Autodesk Fusion 360 part; units mm, degrees
(part 2 of 3)
  line L471 (-71.7601, 16.325) -> (-71.7601, 17.325)
  line L472 (-74.2601, 12.625) -> (-74.2601, 11.625)
  line L473 (-71.1601, 14.475) -> (-70.1601, 13.225) construction
  line L474 (-74.2601, 12.625) -> (-74.2601, 11.625)
  line L475 (-74.8601, 14.475) -> (-75.8601, 13.225) construction
  line L476 (-74.2601, 12.625) -> (-74.2601, 11.625)
  line L477 (-74.2601, 17.325) -> (-73.0101, 16.325) construction
  line L478 (-71.7601, 11.625) -> (-71.7601, 12.625)
  line L479 (-70.1601, 15.725) -> (-71.1601, 15.725)
  line L480 (-74.2601, 11.625) -> (-73.0101, 12.625) construction
  line L481 (-71.7601, 11.625) -> (-71.7601, 12.625)
  line L482 (-75.8601, 15.725) -> (-74.8601, 15.725)
  line L483 (-74.2601, 12.625) -> (-74.2601, 11.625)
  line L484 (-74.8601, 14.475) -> (-75.8601, 13.225) construction
  line L485 (-71.1601, 13.225) -> (-70.1601, 13.225)
  line L486 (-75.8601, 15.725) -> (-74.8601, 15.725)
  line L487 (-74.2601, 12.625) -> (-74.2601, 11.625)
  line L488 (-74.2601, 12.625) -> (-74.2601, 11.625)
  line L489 (-74.2601, 12.625) -> (-74.2601, 11.625)
  line L490 (-74.2601, 17.325) -> (-73.0101, 16.325) construction
  line L491 (-70.1601, 15.725) -> (-71.1601, 15.725)
  line L492 (-75.8601, 15.725) -> (-74.8601, 15.725)
  line L493 (-74.8601, 13.225) -> (-75.8601, 13.225)
  line L494 (-74.8601, 13.225) -> (-75.8601, 13.225)
  line L495 (-75.8601, 15.725) -> (-74.8601, 15.725)
  line L496 (-71.1601, 13.225) -> (-70.1601, 13.225)
  line L497 (-74.8601, 14.475) -> (-75.8601, 13.225) construction
  line L498 (-71.7601, 16.325) -> (-71.7601, 17.325)
  line L499 (-71.1601, 14.475) -> (-70.1601, 13.225) construction
  line L500 (-70.1601, 15.725) -> (-71.1601, 15.725)
  line L501 (-71.1601, 13.225) -> (-70.1601, 13.225)
  line L502 (-74.2601, 17.325) -> (-73.0101, 16.325) construction
  line L503 (-71.1601, 14.475) -> (-70.1601, 13.225) construction
  line L504 (-71.1601, 14.475) -> (-70.1601, 13.225) construction
  line L505 (-74.2601, 17.325) -> (-73.0101, 16.325) construction
  line L506 (-74.2601, 11.625) -> (-73.0101, 12.625) construction
  line L507 (-74.2601, 17.325) -> (-74.2601, 16.325)
  line L508 (-74.8601, 13.225) -> (-75.8601, 13.225)
  line L509 (-70.1601, 15.725) -> (-71.1601, 15.725)
  line L510 (-74.8601, 14.475) -> (-75.8601, 13.225) construction
  line L511 (-71.7601, 11.625) -> (-71.7601, 12.625)
  line L512 (-71.7601, 16.325) -> (-71.7601, 17.325)
  line L513 (-71.7601, 16.325) -> (-71.7601, 17.325)
  line L514 (-71.7601, 11.625) -> (-71.7601, 12.625)
  line L515 (-70.1601, 15.725) -> (-71.1601, 15.725)
  line L516 (-74.2601, 12.625) -> (-74.2601, 11.625)
  line L517 (-74.8601, 13.225) -> (-75.8601, 13.225)
  line L518 (-74.2601, 17.325) -> (-74.2601, 16.325)
  line L519 (-71.7601, 11.625) -> (-71.7601, 12.625)
  line L520 (-74.2601, 17.325) -> (-74.2601, 16.325)
  line L521 (-70.1601, 15.725) -> (-71.1601, 15.725)
  line L522 (-71.1601, 13.225) -> (-70.1601, 13.225)
  line L523 (-71.1601, 13.225) -> (-70.1601, 13.225)
  line L524 (-74.2601, 11.625) -> (-73.0101, 12.625) construction
  line L525 (-70.1601, 15.725) -> (-71.1601, 15.725)
  line L526 (-74.2601, 17.325) -> (-74.2601, 16.325)
  line L527 (-71.7601, 11.625) -> (-71.7601, 12.625)
  line L528 (-71.1601, 13.225) -> (-70.1601, 13.225)
  line L529 (-71.1601, 13.225) -> (-70.1601, 13.225)
  line L530 (-70.1601, 15.725) -> (-71.1601, 14.475) construction
  line L531 (-75.8601, 15.725) -> (-74.8601, 15.725)
  line L532 (-74.2601, 12.625) -> (-74.2601, 11.625)
  line L533 (-74.8601, 13.225) -> (-75.8601, 13.225)
  line L534 (-70.1601, 15.725) -> (-71.1601, 14.475) construction
  line L535 (-75.8601, 15.725) -> (-74.8601, 15.725)
  line L536 (-70.1601, 13.225) -> (-70.1601, 15.725)
  line L537 (-74.8601, 16.325) -> (-74.8601, 12.625)
  line L538 (-70.1601, 13.225) -> (-70.1601, 15.725)
  line L539 (-74.8601, 14.475) -> (-75.8601, 13.225) construction
  line L540 (-74.8601, 14.475) -> (-75.8601, 13.225) construction
  line L541 (-74.2601, 12.625) -> (-74.2601, 11.625)
  line L542 (-75.8601, 15.725) -> (-74.8601, 15.725)
  line L543 (-74.2601, 17.325) -> (-74.2601, 16.325)
  line L544 (-74.2601, 12.625) -> (-74.2601, 11.625)
  line L545 (-74.2601, 12.625) -> (-74.2601, 11.625)
  line L546 (-74.2601, 17.325) -> (-74.2601, 16.325)
  line L547 (-70.1601, 13.225) -> (-70.1601, 15.725)
  line L548 (-75.8601, 15.725) -> (-74.8601, 15.725)
  line L549 (-74.8601, 16.325) -> (-74.8601, 12.625)
  line L550 (-74.2601, 17.325) -> (-73.0101, 16.325) construction
  line L551 (-74.8601, 14.475) -> (-75.8601, 13.225) construction
  line L552 (-74.2601, 17.325) -> (-74.2601, 16.325)
  line L553 (-74.2601, 11.625) -> (-73.0101, 12.625) construction
  line L554 (-70.1601, 15.725) -> (-71.1601, 14.475) construction
  line L555 (-71.1601, 12.625) -> (-71.1601, 16.325)
  line L556 (-74.8601, 13.225) -> (-75.8601, 13.225)
  line L557 (-71.1601, 12.625) -> (-71.1601, 16.325)
  line L558 (-74.2601, 12.625) -> (-74.2601, 11.625)
  line L559 (-70.1601, 13.225) -> (-70.1601, 15.725)
  line L560 (-74.8601, 13.225) -> (-75.8601, 13.225)
  line L561 (-71.1601, 12.625) -> (-71.1601, 16.325)
  line L562 (-70.1601, 15.725) -> (-71.1601, 14.475) construction
  line L563 (-74.8601, 14.475) -> (-75.8601, 13.225) construction
  line L564 (-74.2601, 12.625) -> (-74.2601, 11.625)
  line L565 (-74.2601, 11.625) -> (-73.0101, 12.625) construction
  line L566 (-74.2601, 17.325) -> (-74.2601, 16.325)
  line L567 (-74.2601, 11.625) -> (-73.0101, 12.625) construction
  line L568 (-70.1601, 13.225) -> (-70.1601, 15.725)
  line L569 (-70.1601, 13.225) -> (-70.1601, 15.725)
  line L570 (-74.2601, 17.325) -> (-73.0101, 16.325) construction
  line L571 (-74.8601, 13.225) -> (-75.8601, 13.225)
  line L572 (3.5, 7.3942) -> (-58, 7.3942)
  line L573 (-58, 7.3942) -> (-58, 35.3942)
  line L574 (-58, 35.3942) -> (3.5, 35.3942)
  line L575 (3.5, 35.3942) -> (3.5, 7.3942)
  point P0 (-73.0101, 27.475)
  point P1 (-73.0351, 14.5)
  point P2 (-73.0101, 27.475)
  point P3 (-73.0101, 27.475)
  point P4 (-73.0101, 27.475)
  point P5 (-73.0101, 27.475)
  point P6 (-73.0101, 27.475)
  point P7 (-73.0101, 27.475)
  point P8 (-73.0101, 27.475)
  point P9 (-73.0101, 14.475)
  point P10 (-73.0101, 14.475)
  point P11 (-73.0101, 14.475)
  point P12 (-73.0101, 14.475)
  point P13 (-73.0101, 14.475)
  point P14 (-73.0101, 14.475)
  point P15 (-73.0101, 14.475)
  point P16 (-73.0101, 14.475)
  dimension "d66" = -3
  dimension "d68" = 5
  dimension "d69" = 5
  dimension "d70" = 5
  dimension "d71" = 5
  dimension "d72" = 2
  dimension "d74" = 2
  dimension "d75" = 2
  dimension "d76" = 2
  dimension "d77" = 2
  dimension "d88" = 0.3
  dimension "d122" = 3.7
  dimension "d123" = 3.7
  dimension "d134" = 3.7
  dimension "d135" = 3.7
  dimension "d136" = 3.7
  dimension "d137" = 3.7
  dimension "d138" = 3.7
  dimension "d139" = 3.7
  dimension "d140" = 3.7
  dimension "d141" = 3.7
  dimension "d142" = 3.7
  dimension "d143" = 3.7
  dimension "d144" = 3.7
  dimension "d145" = 3.7
  dimension "d146" = 3.7
  dimension "d147" = 3.7
  dimension "d148" = 3.7
  dimension "d149" = 3.7
  dimension "d150" = 3.7
  dimension "d151" = 3.7
  dimension "d152" = 3.7
  dimension "d153" = 3.7
  dimension "d154" = 3.7
  dimension "d155" = 3.7
  dimension "d156" = 3.7
  dimension "d157" = 3.7
  dimension "d158" = 3.7
  dimension "d159" = 3.7
  dimension "d160" = 3.7
  dimension "d161" = 3.7
  dimension "d162" = 3.7
  dimension "d163" = 3.7
  constraint tangent L18 A12
  constraint tangent L17 A12
  constraint tangent L17 A13
  constraint tangent L16 A13
  constraint tangent L19 A14
  constraint tangent L16 A14
  constraint tangent L18 A15
  constraint tangent L19 A15
  constraint tangent L27 A20
  constraint tangent L26 A20
  constraint tangent L25 A21
  constraint tangent L26 A21
  constraint tangent L24 A22
  constraint tangent L25 A22
  constraint tangent L24 A23
  constraint tangent L27 A23
  constraint horizontal L33
  constraint vertical L34
  constraint horizontal L35
  constraint vertical L36
  constraint coincident L31.end L34.end
  constraint coincident L5.end L6.start
  constraint horizontal L37
  constraint vertical L38
  constraint horizontal L39
  constraint vertical L40
  constraint coincident L4.start L7.end
  constraint coincident L31.start L35.end
  constraint coincident L42 L55.start
  constraint coincident L5 L40.start
  constraint coincident L7 L55.end
  constraint perpendicular L50 L56
  constraint coincident L50 L56.end
  constraint coincident L49 L57.end
  constraint perpendicular L49 L57
  constraint horizontal L58
  constraint perpendicular L58 L59
  constraint parallel L58 L60
  constraint parallel L59 L61
  constraint coincident L62 P8
  constraint coincident L63 P8
  constraint horizontal L64
  constraint perpendicular L64 L68
  constraint parallel L65 L68
  constraint midpoint L60 L66.end
  constraint coincident L60 L68.end
  constraint coincident L60 L65.start
  constraint horizontal L73
  constraint midpoint L59 L70.end
  constraint coincident L59 L72.start
  constraint coincident L59 L73.end
  constraint horizontal L76
  constraint midpoint L61 L75.end
  constraint coincident L61 L76.end
  constraint coincident L61 L77.start
  constraint horizontal L79
  constraint perpendicular L79 L82
  constraint parallel L80 L82
  constraint midpoint L58 L81.end
  constraint coincident L58 L82.end
  constraint coincident L58 L80.start
  constraint horizontal L85
  constraint perpendicular L85 L86
  constraint parallel L84 L86
  constraint horizontal L89
  constraint horizontal L117
  constraint perpendicular L113 L117
  constraint parallel L91 L117
  constraint parallel L110 L113
  constraint coincident P8 L116
  constraint coincident P8 L90
  constraint horizontal L118
  constraint perpendicular L100 L118
  constraint parallel L99 L100
  constraint midpoint L66.end L91
  constraint coincident L68.end L91
  constraint coincident L65.start L91
  constraint horizontal L106
  constraint midpoint L70.end L113
  constraint coincident L72.start L113
  constraint coincident L73.end L113
  constraint horizontal L104
  constraint midpoint L75.end L110
  constraint coincident L76.end L110
  constraint coincident L77.start L110
  constraint horizontal L115
  constraint perpendicular L105 L115
  constraint parallel L105 L111
  constraint midpoint L81.end L117
  constraint coincident L82.end L117
  constraint coincident L80.start L117
  constraint horizontal L119
  constraint perpendicular L114 L119
  constraint parallel L96 L114
  constraint horizontal L102
  constraint midpoint L41 L122.start
  constraint midpoint L43 L122.end
  constraint midpoint L42 L123.start
  constraint midpoint L44 L123.end
  constraint horizontal L158
  constraint perpendicular L151 L158
  constraint parallel L138 L158
  constraint parallel L129 L151
  constraint coincident P8 L164
  constraint coincident P8 L163
  constraint horizontal L140
  constraint perpendicular L140 L149
  constraint parallel L142 L149
  constraint midpoint L66.end L138
  constraint coincident L68.end L138
  constraint coincident L65.start L138
  constraint horizontal L125
  constraint midpoint L70.end L151
  constraint coincident L72.start L151
  constraint coincident L73.end L151
  constraint horizontal L128
  constraint midpoint L75.end L129
  constraint coincident L76.end L129
  constraint coincident L77.start L129
  constraint horizontal L143
  constraint perpendicular L143 L178
  constraint parallel L141 L178
  constraint midpoint L81.end L158
  constraint coincident L82.end L158
  constraint coincident L80.start L158
  constraint horizontal L137
  constraint perpendicular L137 L169
  constraint parallel L169 L186
  constraint horizontal L182
  constraint horizontal L165
  constraint perpendicular L127 L165
  constraint parallel L159 L165
  constraint parallel L127 L174
  constraint coincident P8 L162
  constraint coincident P8 L161
  constraint horizontal L133
  constraint perpendicular L133 L155
  constraint parallel L155 L181
  constraint midpoint L66.end L159
  constraint coincident L68.end L159
  constraint coincident L65.start L159
  constraint horizontal L176
  constraint midpoint L70.end L127
  constraint coincident L72.start L127
  constraint coincident L73.end L127
  constraint horizontal L152
  constraint midpoint L75.end L174
  constraint coincident L76.end L174
  constraint coincident L77.start L174
  constraint horizontal L134
  constraint perpendicular L134 L180
  constraint parallel L157 L180
  constraint midpoint L81.end L165
  constraint coincident L82.end L165
  constraint coincident L80.start L165
  constraint horizontal L136
  constraint perpendicular L124 L136
  constraint parallel L124 L148
  constraint horizontal L175
  constraint horizontal L219
  constraint perpendicular L197 L219
  constraint parallel L219 L226
  constraint parallel L197 L198
  constraint coincident P8 L212
  constraint coincident P8 L215
  constraint horizontal L191
  constraint perpendicular L191 L283
  constraint parallel L252 L283
  constraint midpoint L66.end L226
  constraint coincident L68.end L226
  constraint coincident L65.start L226
  constraint horizontal L262
  constraint midpoint L70.end L197
  constraint coincident L72.start L197
  constraint coincident L73.end L197
  constraint horizontal L246
  constraint midpoint L75.end L198
  constraint coincident L76.end L198
  constraint coincident L77.start L198
  constraint horizontal L216
  constraint perpendicular L216 L248
  constraint parallel L238 L248
  constraint midpoint L81.end L219
  constraint coincident L82.end L219
  constraint coincident L80.start L219
  constraint horizontal L221
  constraint perpendicular L221 L258
  constraint parallel L251 L258
  constraint horizontal L291
  constraint horizontal L218
  constraint perpendicular L218 L228
  constraint parallel L218 L220
  constraint parallel L196 L228
  constraint coincident P8 L217
  constraint coincident P8 L213
  constraint horizontal L225
  constraint perpendicular L225 L242
  constraint parallel L242 L300
  constraint midpoint L66.end L220
  constraint coincident L68.end L220
  constraint coincident L65.start L220
  constraint horizontal L247
  constraint midpoint L70.end L228
  constraint coincident L72.start L228
  constraint coincident L73.end L228
  constraint horizontal L268
  constraint midpoint L75.end L196
  constraint coincident L76.end L196
  constraint coincident L77.start L196
  constraint horizontal L188
  constraint perpendicular L188 L233
  constraint parallel L233 L264
  constraint midpoint L81.end L218
  constraint coincident L82.end L218
  constraint coincident L80.start L218
  constraint horizontal L224
  constraint perpendicular L224 L260
  constraint parallel L260 L314
  constraint horizontal L234
  constraint horizontal L194
  constraint perpendicular L194 L239
  constraint parallel L194 L206
  constraint parallel L239 L261
  constraint coincident P8 L203
  constraint coincident P8 L202
  constraint horizontal L214
  constraint perpendicular L214 L292
  constraint parallel L292 L299
  constraint midpoint L66.end L206
  constraint coincident L68.end L206
  constraint coincident L65.start L206
  constraint horizontal L280
  constraint midpoint L70.end L239
  constraint coincident L72.start L239
  constraint coincident L73.end L239
  constraint horizontal L296
  constraint midpoint L75.end L261
  constraint coincident L76.end L261
  constraint coincident L77.start L261
  constraint horizontal L192
  constraint perpendicular L192 L272
  constraint parallel L272 L276
  constraint midpoint L81.end L194
  constraint coincident L82.end L194
  constraint coincident L80.start L194
  constraint horizontal L193
  constraint perpendicular L193 L290
  constraint parallel L278 L290
  constraint horizontal L282
  constraint horizontal L195
  constraint perpendicular L195 L229
  constraint parallel L195 L210
  constraint parallel L229 L243
  constraint coincident P8 L204
  constraint coincident P8 L201
  constraint horizontal L207
  constraint perpendicular L207 L293
  constraint parallel L293 L312
  constraint midpoint L66.end L210
  constraint coincident L68.end L210
  constraint coincident L65.start L210
  constraint horizontal L240
  constraint midpoint L70.end L229
  constraint coincident L72.start L229
  constraint coincident L73.end L229
  constraint horizontal L286
  constraint midpoint L75.end L243
  constraint coincident L76.end L243
  constraint coincident L77.start L243
  constraint horizontal L200
  constraint perpendicular L200 L304
  constraint parallel L294 L304
  constraint midpoint L81.end L195
  constraint coincident L82.end L195
  constraint coincident L80.start L195
  constraint horizontal L205
  constraint perpendicular L205 L288
  constraint parallel L285 L288
  constraint horizontal L311
  constraint horizontal L348
  constraint perpendicular L348 L357
  constraint parallel L317 L348
  constraint parallel L357 L369
  constraint coincident P16 L340
  constraint coincident P16 L327
  constraint horizontal L423
  constraint perpendicular L423 L514
  constraint parallel L488 L514
  constraint midpoint L319.end L317
  constraint coincident L431.end L317
  constraint coincident L440.start L317
  constraint horizontal L548
  constraint midpoint L351.end L357
  constraint coincident L493.start L357
  constraint coincident L482.end L357
  constraint horizontal L515
  constraint midpoint L361.end L369
  constraint coincident L433.end L369
  constraint coincident L435.start L369
  constraint horizontal L346
  constraint perpendicular L346 L546
  constraint parallel L463 L546
  constraint midpoint L326.end L348
  constraint coincident L507.end L348
  constraint coincident L429.start L348
  constraint horizontal L337
  constraint perpendicular L337 L481
  constraint parallel L481 L564
  constraint horizontal L525
  constraint horizontal L424
  constraint perpendicular L385 L424
  constraint parallel L338 L424
  constraint parallel L350 L385
  constraint coincident P16 L341
  constraint coincident P16 L342
  constraint horizontal L344
  constraint perpendicular L344 L519
  constraint parallel L519 L544
  constraint midpoint L319.end L338
  constraint coincident L431.end L338
  constraint coincident L440.start L338
  constraint horizontal L542
  constraint midpoint L351.end L385
  constraint coincident L493.start L385
  constraint coincident L482.end L385
  constraint horizontal L443
  constraint midpoint L361.end L350
  constraint coincident L433.end L350
  constraint coincident L435.start L350
  constraint horizontal L425
  constraint perpendicular L425 L566
  constraint parallel L512 L566
  constraint midpoint L326.end L424
  constraint coincident L507.end L424
  constraint coincident L429.start L424
  constraint horizontal L426
  constraint perpendicular L426 L527
  constraint parallel L527 L532
  constraint horizontal L509
  constraint horizontal L427
  constraint perpendicular L353 L427
  constraint parallel L325 L427
  constraint parallel L353 L368
  constraint coincident P16 L334
  constraint coincident P16 L339
  constraint horizontal L345
  constraint perpendicular L345 L444
  constraint parallel L444 L545
  constraint midpoint L319.end L325
  constraint coincident L431.end L325
  constraint coincident L440.start L325
  constraint horizontal L531
  constraint midpoint L351.end L353
  constraint coincident L493.start L353
  constraint coincident L482.end L353
  constraint horizontal L500
  constraint midpoint L361.end L368
  constraint coincident L433.end L368
  constraint coincident L435.start L368
  constraint horizontal L320
  constraint perpendicular L320 L543
  constraint parallel L498 L543
  constraint midpoint L326.end L427
  constraint coincident L507.end L427
  constraint coincident L429.start L427
  constraint horizontal L343
  constraint perpendicular L343 L478
  constraint parallel L478 L558
  constraint horizontal L479
  constraint horizontal L347
  constraint perpendicular L347 L366
  constraint parallel L329 L347
  constraint parallel L360 L366
  constraint coincident P16 L322
  constraint coincident P16 L321
  constraint horizontal L333
  constraint perpendicular L333 L511
  constraint parallel L483 L511
  constraint midpoint L319.end L329
  constraint coincident L431.end L329
  constraint coincident L440.start L329
  constraint horizontal L535
  constraint midpoint L351.end L366
  constraint coincident L493.start L366
  constraint coincident L482.end L366
  constraint horizontal L521
  constraint midpoint L361.end L360
  constraint coincident L433.end L360
  constraint coincident L435.start L360
  constraint horizontal L328
  constraint perpendicular L328 L552
  constraint parallel L513 L552
  constraint midpoint L326.end L347
  constraint coincident L507.end L347
  constraint coincident L429.start L347
  constraint horizontal L316
  constraint perpendicular L316 L436
  constraint parallel L436 L541
  constraint horizontal L491
  constraint horizontal L409
  constraint perpendicular L409 L549
  constraint parallel L402 L409
  constraint parallel L549 L555
  constraint coincident P16 L406
  constraint coincident P16 L394
  constraint horizontal L412
  constraint perpendicular L412 L459
  constraint parallel L459 L474
  constraint midpoint L319.end L402
  constraint coincident L431.end L402
  constraint coincident L440.start L402
  constraint horizontal L482
  constraint midpoint L351.end L549
  constraint coincident L493.start L549
  constraint coincident L482.end L549
  constraint horizontal L434
  constraint midpoint L361.end L555
  constraint coincident L433.end L555
  constraint coincident L435.start L555
  constraint horizontal L405
  constraint perpendicular L405 L526
  constraint parallel L462 L526
  constraint midpoint L326.end L409
  constraint coincident L507.end L409
  constraint coincident L429.start L409
  constraint horizontal L330
  constraint perpendicular L330 L449
  constraint parallel L449 L476
  constraint horizontal L453
  constraint horizontal L392
  constraint perpendicular L359 L392
  constraint parallel L392 L395
  constraint parallel L352 L359
  constraint coincident P16 L413
  constraint coincident P16 L404
  constraint horizontal L318
  constraint perpendicular L318 L458
  constraint parallel L458 L489
  constraint midpoint L319.end L395
  constraint coincident L431.end L395
  constraint coincident L440.start L395
  constraint horizontal L492
  constraint midpoint L351.end L359
  constraint coincident L493.start L359
  constraint coincident L482.end L359
  constraint horizontal L438
  constraint midpoint L361.end L352
  constraint coincident L433.end L352
  constraint coincident L435.start L352
  constraint horizontal L408
  constraint perpendicular L408 L507
  constraint parallel L471 L507
  constraint midpoint L326.end L392
  constraint coincident L507.end L392
  constraint coincident L429.start L392
  constraint horizontal L421
  constraint perpendicular L421 L441
  constraint parallel L441 L516
  constraint horizontal L433
  constraint horizontal L397
  constraint perpendicular L386 L397
  constraint parallel L397 L416
  constraint parallel L386 L557
  constraint coincident P16 L414
  constraint coincident P16 L389
  constraint horizontal L401
  constraint perpendicular L401 L437
  constraint parallel L437 L472
  constraint midpoint L319.end L416
  constraint coincident L431.end L416
  constraint coincident L440.start L416
  constraint horizontal L495
  constraint midpoint L351.end L386
  constraint coincident L493.start L386
  constraint coincident L482.end L386
  constraint horizontal L461
  constraint midpoint L361.end L557
  constraint coincident L433.end L557
  constraint coincident L435.start L557
  constraint horizontal L399
  constraint perpendicular L399 L518
  constraint parallel L430 L518
  constraint midpoint L326.end L397
  constraint coincident L507.end L397
  constraint coincident L429.start L397
  constraint horizontal L422
  constraint perpendicular L422 L457
  constraint parallel L457 L487
  constraint horizontal L448
  constraint horizontal L420
  constraint perpendicular L420 L537
  constraint parallel L400 L420
  constraint parallel L537 L561
  constraint coincident P16 L390
  constraint coincident P16 L410
  constraint horizontal L403
  constraint perpendicular L403 L467
  constraint parallel L440 L467
  constraint midpoint L319.end L400
  constraint coincident L431.end L400
  constraint coincident L440.start L400
  constraint horizontal L486
  constraint midpoint L351.end L537
  constraint coincident L493.start L537
  constraint coincident L482.end L537
  constraint horizontal L460
  constraint midpoint L361.end L561
  constraint coincident L433.end L561
  constraint coincident L435.start L561
  constraint horizontal L418
  constraint perpendicular L418 L520
  constraint parallel L429 L520
  constraint midpoint L326.end L420
  constraint coincident L507.end L420
  constraint coincident L429.start L420
  constraint horizontal L393
  constraint perpendicular L393 L431
  constraint parallel L431 L466
  constraint horizontal L470
  measures "d68" radius of A12
  measures "d69" radius of A13
  measures "d70" radius of A14
  measures "d71" radius of A15
  measures "d74" radius of A20
  measures "d75" radius of A21
  measures "d76" radius of A22
  measures "d77" radius of A23
  measures "d122" distance of L59.end L60.end
  measures "d123" distance of L58.end L59.end
  measures "d134" distance of L60.end L59.end
  measures "d135" distance of L58.end L59.end
  measures "d136" distance of L60.end L59.end
  measures "d137" distance of L58.end L59.end
  measures "d138" distance of L60.end L59.end
  measures "d139" distance of L58.end L59.end
  measures "d140" distance of L60.end L59.end
  measures "d141" distance of L58.end L59.end
  measures "d142" distance of L60.end L59.end
  measures "d143" distance of L58.end L59.end
  measures "d144" distance of L60.end L59.end
  measures "d145" distance of L59.end L58.end
  measures "d146" distance of L59.end L60.end
  measures "d147" distance of L59.end L58.end
  measures "d148" distance of L317.end L317.start
  measures "d149" distance of L321.start L317.start
  measures "d150" distance of L317.end L317.start
  measures "d151" distance of L321.start L317.start
  measures "d152" distance of L317.end L317.start
  measures "d153" distance of L317.start L321.start
  measures "d154" distance of L317.start L317.end
  measures "d155" distance of L317.start L321.start
  measures "d156" distance of L317.start L317.end
  measures "d157" distance of L317.start L321.start
  measures "d158" distance of L317.end L317.start
  measures "d159" distance of L321.start L317.start
  measures "d160" distance of L317.end L317.start
  measures "d161" distance of L317.start L321.start
  measures "d162" distance of L317.start L317.end
  measures "d163" distance of L317.start L321.start
extrude "Extrude10" cut sketch "Sketch4" against normal blind 0.5 contours A8 L12 A9 L13 A10 L14 A11 L15 | L16 L17 L18 L19 A12 A13 A14 A15 | L24 L25 L26 L27 A20 A21 A22 A23 bodies 2
extrude "Extrude11" add sketch "Sketch4" against normal blind 0.5 separate body contours A0 L0 A1 L1 A2 L2 A3 L3 | A8 L12 A9 L13 A10 L14 A11 L15 | L16 L17 L18 L19 A12 A13 A14 A15 makes body 3 at (-1.3333, 56.6667, 20) makes body 4 at (30.3333, -9.8109, 20)
extrude "Extrude12" add sketch "Sketch1" along normal blind 14 from surface at 2 separate body contours L0 L1 L2 L3 A0 A1 A2 A3 L59 L63 L68 L72 makes body 5
extrude "Extrude13" add sketch "Sketch4" against normal blind 2 from surface at -0.5 separate body contours L24 L25 L26 L27 A20 A21 A22 A23 makes body 6
extrude "Extrude14" add sketch "Sketch4" against normal blind 2 from surface at -4 separate body contours L4 L5 L7 L28 L29 L30 L38 L39 L40 L49 L50 L52 L53 L54 L56 L57 | L4 L5 L7 L28 L29 L30 L31 L35 L37 L38 L39 L40 | L45 L46 L47 L48 | L58 L59 L60 L61 L91 L110 L113 L117 L127 L129 L138 L151 L158 L159 L165 L174 L194 L195 L196 L197 L198 L206 L210 L218 L219 L220 L226 L228 L229 L239 L243 L261 | L58 L79 L80 L82 L105 L111 L115 L117 L134 L141 L143 L157 L158 L165 L178 L180 L188 L192 L194 L195 L200 L216 L218 L219 L233 L238 L248 L264 L272 L276 L294 L304 | L61 L74 L76 L77 L87 L88 L89 L92 L97 L102 L104 L107 L109 L110 L128 L129 L131 L150 L152 L170 L172 L173 L174 L175 L177 L182 L184 L187 L196 L198 L227 L230 L232 L234 L237 L241 L243 L246 L250 L254 L256 L261 L266 L268 L282 L286 L289 L291 L296 L297 L298 L301 L303 L306 L307 L311 | L59 L69 L72 L73 L103 L106 L108 L113 L125 L127 L130 L132 L151 L160 L167 L176 L197 L228 L229 L236 L239 L240 L247 L253 L255 L262 L270 L271 L279 L280 L284 L295 | L60 L64 L65 L68 L84 L85 L86 L91 L96 L99 L100 L114 L118 L119 L124 L133 L136 L137 L138 L140 L142 L148 L149 L155 L159 L169 L181 L186 L191 L193 L205 L206 L207 L210 L214 L220 L221 L224 L225 L226 L242 L251 L252 L258 L260 L278 L283 L285 L288 L290 L292 L293 L299 L300 L312 L314 makes body 7
extrude "Extrude15" add sketch "Sketch4" against normal blind 2 from surface at -4 separate body contours L5 L6 L7 L28 L29 L31 L32 L33 L34 L35 L36 L37 | L5 L6 L7 L28 L29 L32 L33 L34 L36 L49 L50 L51 L56 L57 | L41 L42 L43 L44 | L316 L317 L318 L325 L329 L330 L333 L337 L338 L343 L344 L345 L393 L395 L400 L401 L402 L403 L412 L416 L421 L422 L423 L426 L431 L436 L437 L440 L441 L444 L449 L457 L458 L459 L466 L467 L472 L474 L476 L478 L481 L483 L487 L488 L489 L511 L514 L516 L519 L527 L532 L541 L544 L545 L558 L564 | L317 L325 L329 L338 L347 L348 L350 L352 L353 L357 L359 L360 L366 L368 L369 L385 L386 L392 L395 L397 L400 L402 L409 L416 L420 L424 L427 L537 L549 L555 L557 L561 | L353 L355 L357 L358 L359 L364 L366 L367 L371 L375 L378 L383 L385 L386 L482 L486 L492 L493 L494 L495 L508 L517 L531 L533 L535 L537 L542 L548 L549 L556 L560 L571 | L349 L350 L352 L356 L360 L362 L365 L368 L369 L377 L379 L380 L384 L388 L391 L433 L434 L435 L438 L439 L443 L445 L446 L447 L448 L450 L451 L452 L453 L454 L460 L461 L470 L479 L485 L491 L496 L500 L501 L509 L515 L521 L522 L523 L525 L528 L529 L536 L538 L547 L555 L557 L559 L561 L568 L569 | L320 L328 L346 L347 L348 L392 L397 L399 L405 L408 L409 L418 L420 L424 L425 L427 L429 L430 L462 L463 L471 L498 L507 L512 L513 L518 L520 L526 L543 L546 L552 L566 makes body 8
extrude "Extrude16" add sketch "Sketch4" against normal blind 5 from surface at 1 contours L41 L42 L43 L44 | L316 L317 L318 L325 L329 L330 L333 L337 L338 L343 L344 L345 L393 L395 L400 L401 L402 L403 L412 L416 L421 L422 L423 L426 L431 L436 L437 L440 L441 L444 L449 L457 L458 L459 L466 L467 L472 L474 L476 L478 L481 L483 L487 L488 L489 L511 L514 L516 L519 L527 L532 L541 L544 L545 L558 L564 | L317 L325 L329 L338 L347 L348 L350 L352 L353 L357 L359 L360 L366 L368 L369 L385 L386 L392 L395 L397 L400 L402 L409 L416 L420 L424 L427 L537 L549 L555 L557 L561 | L353 L355 L357 L358 L359 L364 L366 L367 L371 L375 L378 L383 L385 L386 L482 L486 L492 L493 L494 L495 L508 L517 L531 L533 L535 L537 L542 L548 L549 L556 L560 L571 | L349 L350 L352 L356 L360 L362 L365 L368 L369 L377 L379 L380 L384 L388 L391 L433 L434 L435 L438 L439 L443 L445 L446 L447 L448 L450 L451 L452 L453 L454 L460 L461 L470 L479 L485 L491 L496 L500 L501 L509 L515 L521 L522 L523 L525 L528 L529 L536 L538 L547 L555 L557 L559 L561 L568 L569 | L320 L328 L346 L347 L348 L392 L397 L399 L405 L408 L409 L418 L420 L424 L425 L427 L429 L430 L462 L463 L471 L498 L507 L512 L513 L518 L520 L526 L543 L546 L552 L566 bodies 8
extrude "Extrude17" add sketch "Sketch4" against normal blind 5 from surface at 1 contours L45 L46 L47 L48 | L58 L59 L60 L61 L91 L110 L113 L117 L127 L129 L138 L151 L158 L159 L165 L174 L194 L195 L196 L197 L198 L206 L210 L218 L219 L220 L226 L228 L229 L239 L243 L261 | L58 L79 L80 L82 L105 L111 L115 L117 L134 L141 L143 L157 L158 L165 L178 L180 L188 L192 L194 L195 L200 L216 L218 L219 L233 L238 L248 L264 L272 L276 L294 L304 | L61 L74 L76 L77 L87 L88 L89 L92 L97 L102 L104 L107 L109 L110 L128 L129 L131 L150 L152 L170 L172 L173 L174 L175 L177 L182 L184 L187 L196 L198 L227 L230 L232 L234 L237 L241 L243 L246 L250 L254 L256 L261 L266 L268 L282 L286 L289 L291 L296 L297 L298 L301 L303 L306 L307 L311 | L59 L69 L72 L73 L103 L106 L108 L113 L125 L127 L130 L132 L151 L160 L167 L176 L197 L228 L229 L236 L239 L240 L247 L253 L255 L262 L270 L271 L279 L280 L284 L295 | L60 L64 L65 L68 L84 L85 L86 L91 L96 L99 L100 L114 L118 L119 L124 L133 L136 L137 L138 L140 L142 L148 L149 L155 L159 L169 L181 L186 L191 L193 L205 L206 L207 L210 L214 L220 L221 L224 L225 L226 L242 L251 L252 L258 L260 L278 L283 L285 L288 L290 L292 L293 L299 L300 L312 L314 bodies 7
chamfer "Chamfer1" distance 1 angle 45 4 edges at (66.8351, -14.5, 21) (73.0351, -20.7, 21) (73.0351, -8.3, 21) (79.2351, -14.5, 21) on bodies 8
chamfer "Chamfer2" distance 1 angle 45 4 edges at (73.0351, -21.3, 21) (66.8351, -27.5, 21) (73.0351, -33.7, 21) (79.2351, -27.5, 21) on bodies 7
fillet "Fillet3" radius 1 8 edges at (73.0351, -22.3, 21) (67.8351, -27.5, 21) (73.0351, -32.7, 21) (78.2351, -27.5, 21) (73.0351, -9.3, 21) (67.8351, -14.5, 21) (73.0351, -19.7, 21) (78.2351, -14.5, 21) on bodies 7 8
extrude "Extrude18" add sketch "Sketch3" along normal blind 6 from surface at -4 separate body contours A1 makes body 9
fillet "Fillet4" radius 1 1 edges at (96, 52.4527, 6.8484) on bodies 9
extrude "Extrude19" add sketch "Sketch3" along normal blind 6 from surface at -112 separate body contours A1 makes body 10
fillet "Fillet5" radius 1 1 faces at (-18, 57.0083, 7.2824) on bodies 10
ref_plane "WorkPlane2" through (39, 65.5, 16.5) normal (0, 0, 1) x (1, 0, 0)
split "Split2" by plane through (39, 65.5, 16.5) normal (0, 0, 1) bodies 2 makes body 11 at (89, 41.6667, 20)
extrude "Extrude20" add sketch "Sketch1" against normal blind 3 from surface at 16.5 contours L41 L44 L48 L49 L51 L78 | L41 L49 L75 L76 L77 L78 L99 | L41 L49 L76 L94 | L43 L44 L47 L48 L52 L90 | L41 L49 L91 L92 L93 L94 L103 | L41 L49 L84 L92 | L43 L47 L87 L88 L89 L90 L107 | L41 L49 L83 L84 L85 L86 L119 | L43 L47 L88 L98 | L41 L42 L49 L50 L54 L86 | L43 L47 L95 L96 L97 L98 L115 | L43 L47 L80 L96 | L43 L47 L79 L80 L81 L82 L111 | L42 L43 L47 L50 L53 L82 bodies 2
extrude "Extrude21" cut sketch "Sketch1" against normal blind 3 from surface at 20 contours L20 L21 A21 | L20 A21 | L22 A23 | L21 L22 A23 | L21 A21 | L21 A23 | A8 | A10 | A12 | A13 | A15 | A16 | A18 | A19 | A22 | A24 | A26 | A27 | A28 | A29 | A30 | A31 picked at (-10.6507, -35.0016) picked at (83.9483, -39.6079) bodies 11
extrude "Extrude22" cut sketch "Sketch1" along normal blind 35 contours A10 | A13 | A16 | A19 | A22 | A24 bodies 2
extrude "Extrude23" cut sketch "Sketch1" along normal blind 13 contours A24 | A30 bodies 1
chamfer "Chamfer3" distance 2 angle 45 1 edges at (83.4223, -37.994, 0) on bodies 1
extrude "Extrude24" cut sketch "Sketch1" along normal blind 13 contours A10 | A13 | A16 | A19 | A22 | A26 | A27 | A28 | A29 | A31 bodies 1 2
chamfer "Chamfer4" distance 2 angle 45 5 edges at (-5.2918, 161.7335, 0) (78.1641, 161.7335, 0) (-10.5777, 79.006, 0) (83.4223, 79.006, 0) (-10.5777, -37.994, 0) on bodies 1
extrude "Extrude25" cut sketch "Sketch1" against normal blind 15 from surface at 17 contours L0 L19 L59 L60 L61 L62 L63 L64 bodies 2
extrude "Extrude26" cut sketch "Sketch1" along normal blind 35 contours A10 | A13 | A16 | A19 | A22 | A24 | A26 | A27 | A28 | A29 | A30 | A31 bodies 2
extrude "Extrude27" cut sketch "Sketch1" along normal blind 40 contours A10 | A13 | A16 | A19 | A22 | A24 | A26 | A27 | A28 | A29 | A30 | A31 bodies 11
extrude "Extrude28" cut sketch "Sketch1" along normal blind 20 contours L3 L65 L66 L67 L68 | L1 L69 L70 L71 L72 bodies 2
ref_plane "WorkPlane4" through (39, 114, 10) normal (0, -1, 0) x (1, 0, 0)
split "Split3" by plane through (39, 114, 10) normal (0, -1, 0) bodies 2 makes body 12 at (-8.8305, 17.9357, 16.5)
split "Split4" by plane through (39, 114, 10) normal (0, -1, 0) bodies 1 makes body 13 at (54.0813, 2.7171, 2)
split "Split5" by plane through (39, 114, 10) normal (0, -1, 0) bodies 3 makes body 14 at (0.3333, 44.6667, 20)
split "Split6" by plane through (39, 114, 10) normal (0, -1, 0) bodies 11 makes body 15 at (-8.8305, 17.9357, 16.5)
sketch "Sketch5" plane through (0, 114, 0) normal (0, 1, 0) x (-1, 0, 0)
  line L0 (-80, 2) -> (-80, 16.5)
  line L1 (-80, 16.5) -> (-94, 16.5)
  line L2 (-94, 16.5) -> (-94, 2)
  line L3 (-94, 2) -> (-80, 2)
  line L4 (2, 16.5) -> (2, 2)
  line L5 (2, 2) -> (16, 2)
  line L6 (16, 2) -> (16, 16.5)
  line L7 (16, 16.5) -> (2, 16.5)
  line L8 (-93, 15.5) -> (-93, 3)
  line L9 (-93, 3) -> (-81, 3)
  line L10 (-81, 3) -> (-81, 15.5)
  line L11 (15, 3) -> (15, 15.5)
  line L12 (3, 15.5) -> (3, 3)
  line L13 (3, 3) -> (15, 3)
  line L14 (-93.2, 15.7) -> (-93.2, 2.8)
  line L15 (-93.2, 2.8) -> (-80.8, 2.8)
  line L16 (-80.8, 2.8) -> (-80.8, 15.7)
  line L17 (15.2, 2.8) -> (15.2, 15.7)
  line L18 (2.8, 15.7) -> (2.8, 2.8)
  line L19 (2.8, 2.8) -> (15.2, 2.8)
  line L20 (-93.2, 15.7) -> (-93.2, 16.5)
  line L21 (-93, 15.5) -> (-93, 16.5)
  line L22 (-80.8, 15.7) -> (-80.8, 16.5)
  line L23 (-81, 15.5) -> (-81, 16.5)
  line L24 (2.8, 15.7) -> (2.8, 16.5)
  line L25 (3, 15.5) -> (3, 16.5)
  line L26 (15.2, 15.7) -> (15.2, 16.5)
  line L27 (15, 15.5) -> (15, 16.5)
  constraint coincident L1 L20.end
  constraint perpendicular L1 L20
  constraint coincident L1 L21.end
  constraint perpendicular L1 L21
  constraint coincident L1 L22.end
  constraint perpendicular L1 L22
  constraint coincident L1 L23.end
  constraint perpendicular L1 L23
  constraint coincident L7 L24.end
  constraint perpendicular L7 L24
  constraint coincident L7 L25.end
  constraint perpendicular L7 L25
  constraint coincident L7 L26.end
  constraint perpendicular L7 L26
  constraint coincident L7 L27.end
  constraint perpendicular L7 L27
extrude "Extrude29" add sketch "Sketch5" along normal blind 15 contours L1 L8 L9 L10 L21 L23 bodies 12
extrude "Extrude30" add sketch "Sketch5" along normal blind 15 contours L7 L11 L12 L13 L25 L27 bodies 12
extrude "Extrude31" cut sketch "Sketch5" along normal blind 15.3 contours L7 L11 L12 L13 L17 L18 L19 L24 L25 L26 L27 | L7 L11 L12 L13 L25 L27 bodies 2
extrude "Extrude32" cut sketch "Sketch5" along normal blind 15.3 contours L1 L8 L9 L10 L14 L15 L16 L20 L21 L22 L23 | L1 L8 L9 L10 L21 L23 bodies 2
sketch "Sketch6" plane through (0, 0, 2) normal (0, 0, 1) x (-1, 0, 0)
  line L0 (-94, -114) -> (16, -114)
  line L1 (16, -114) -> (16, 35)
  arc A0 (16, 35) -> (6, 45) centre (6, 35) ccw
  line L2 (6, 45) -> (-84, 45)
  arc A1 (-84, 45) -> (-94, 35) centre (-84, 35) ccw
  line L3 (-94, 35) -> (-94, -114)
  circle A2 centre (-85.9862, 36.9996) radius 2.75
  circle A3 centre (8.0138, 36.9996) radius 2.75
  circle A4 centre (8.0138, -80.0004) radius 2.75
  circle A5 centre (-85.9862, -80.0004) radius 2.75
  line L4 (16, -114) -> (-94, -114)
  line L5 (-94, -114) -> (-94, -150)
  arc A6 (-94, -150) -> (-68, -176) centre (-68, -150) ccw
  line L6 (-68, -176) -> (-10, -176)
  arc A7 (-10, -176) -> (16, -150) centre (-10, -150) ccw
  line L7 (16, -150) -> (16, -114)
  circle A8 centre (-80.728, -162.7279) radius 2.75
  circle A9 centre (2.7279, -162.7279) radius 2.75
  line L8 (0, -65.7044) -> (-5, -65.7044)
  line L9 (-78, -89.1708) -> (-78, -10)
  line L10 (-78, -65.7044) -> (-73, -65.7044)
  line L11 (-5, -111.4785) -> (-73, -111.4785)
  line L12 (-73, -111.4785) -> (-73, -6.0753)
  line L13 (-73, -6.0753) -> (-5, -6.0753)
  line L14 (-5, -6.0753) -> (-5, -111.4785)
  line L15 (-31, -116.9153) -> (-5.271, -116.9153)
  line L16 (-5.271, -116.9153) -> (-5.271, -155.1481)
  line L17 (-5.271, -155.1481) -> (-31, -155.1481)
  line L18 (-31, -155.1481) -> (-31, -116.9153)
  dimension "d236" = 5
  dimension "d237" = 5
  constraint horizontal L8
  constraint coincident L9 L10.start
  constraint perpendicular L9 L10
  constraint horizontal L11
  constraint vertical L12
  constraint horizontal L13
  constraint vertical L14
  constraint horizontal L15
  constraint vertical L16
  constraint horizontal L17
  constraint vertical L18
  measures "d236" distance of L8.start L8.end
  measures "d237" distance of L10.start L10.end
extrude "Extrude33" add sketch "Sketch6" along normal blind 6 contours L15 L16 L17 L18 bodies 1
extrude "Extrude34" add sketch "Sketch6" along normal blind 6 contours L11 L12 L13 L14 bodies 13
fillet "Fillet6" radius 2.5 8 edges at (5.271, 136.0317, 8) (18.1355, 116.9153, 8) (31, 136.0317, 8) (18.1355, 155.1481, 8) (73, 58.7769, 8) (39, 6.0753, 8) (5, 58.7769, 8) (39, 111.4785, 8) on bodies 1 13
extrude "Extrude50" add sketch "Sketch1" against normal blind 1 from surface at 13.5 contours L41 L49 L75 L76 L77 L78 L99 | L41 L49 L91 L92 L93 L94 L103 | L43 L47 L87 L88 L89 L90 L107 | L41 L49 L83 L84 L85 L86 L119 | L43 L47 L95 L96 L97 L98 L115 | L43 L47 L79 L80 L81 L82 L111 bodies 12
extrude "Extrude36" add sketch "Sketch1" against normal blind 1 from surface at 13.5 contours L41 L77 L99 L100 L101 L102 | L41 L91 L103 L104 L105 L106 | L43 L87 L107 L108 L109 L110 | L41 L83 L119 L120 L121 L122 | L43 L97 L115 L116 L117 L118 | L43 L81 L111 L112 L113 L114 bodies 12
sketch "Sketch7" plane through (0, 0, 16) normal (0, 0, -1) x (1, 0, 0)
  circle A0 centre (-8.0138, 36.9996) radius 2.75
  circle A1 centre (85.9862, 36.9996) radius 2.75
  line L0 (66.5351, 34) -> (79.5351, 34)
  line L1 (79.5351, 34) -> (79.5351, 8)
  line L2 (79.5351, 8) -> (66.5351, 8)
  line L3 (66.5351, 8) -> (66.5351, 34)
  line L4 (58, 7.3942) -> (-3.5, 7.3942)
  line L5 (-3.5, 7.3942) -> (-3.5, 12.982)
  line L6 (-3.5, 12.982) -> (-3.5, 26.0298)
  line L7 (-3.5, 26.0298) -> (-3.5, 35.3942)
  line L8 (-3.5, 35.3942) -> (58, 35.3942)
  line L9 (58, 35.3942) -> (58, 26.0298)
  line L10 (58, 26.0298) -> (58, 12.982)
  line L11 (58, 12.982) -> (58, 7.3942)
  line L12 (89, -38) -> (89, 40)
  line L13 (89, 40) -> (-11, 40)
  line L14 (-11, 40) -> (-11, -38)
  line L15 (-11, -38) -> (-15, -38)
  line L16 (-15, -38) -> (-15, -66)
  line L17 (-15, -66) -> (-2, -66)
  line L18 (-2, -66) -> (-2, -38)
  line L19 (-2, -38) -> (-6, -38)
  line L20 (-6, -38) -> (-6, 4)
  line L21 (-6, 4) -> (31.5, 4)
  line L22 (84, 4) -> (84, -38)
  line L23 (84, -38) -> (80, -38)
  line L24 (80, -38) -> (80, -66)
  line L25 (80, -66) -> (93, -66)
  line L26 (93, -66) -> (93, -38)
  line L27 (93, -38) -> (89, -38)
  line L28 (19.8248, 8.3942) -> (19.8248, 9.8942)
  line L29 (29.8248, 9.8942) -> (29.8248, 8.3942)
  line L30 (3.562, 9.8942) -> (3.562, 8.3942)
  line L31 (-1.438, 8.3942) -> (-1.438, 9.8942)
  line L32 (-1.438, 32.8942) -> (-1.438, 34.3942)
  line L33 (3.562, 34.3942) -> (3.562, 32.8942)
  line L34 (19.8248, 32.8942) -> (19.8248, 34.3942)
  line L35 (29.8248, 34.3942) -> (29.8248, 32.8942)
  line L36 (19.8348, 4) -> (3.562, 4)
  line L37 (3.562, 4) -> (3.562, 7.3942)
  line L38 (3.562, 9.8942) -> (19.8348, 9.8942)
  line L39 (19.8348, 9.8942) -> (19.8348, 4)
  line L40 (3.662, 4.1) -> (3.662, 9.7942)
  line L41 (3.662, 9.7942) -> (19.7348, 9.7942)
  line L42 (19.7348, 9.7942) -> (19.7348, 4.1)
  line L43 (19.7348, 4.1) -> (3.662, 4.1)
  line L44 (19.8248, 32.8942) -> (3.562, 32.8942)
  line L45 (3.562, 32.8942) -> (3.562, 40)
  line L46 (3.562, 40) -> (19.8248, 40)
  line L47 (19.8248, 40) -> (19.8248, 35.3942)
  line L48 (19.7248, 39.9) -> (19.7248, 32.9942)
  line L49 (19.7248, 32.9942) -> (3.662, 32.9942)
  line L50 (3.662, 32.9942) -> (3.662, 39.9)
  line L51 (3.662, 39.9) -> (19.7248, 39.9)
  line L52 (19.7348, 9.7942) -> (3.662, 9.7942)
  line L53 (3.662, 9.7942) -> (3.662, 32.9942)
  line L54 (3.662, 32.9942) -> (19.7348, 32.9942)
  line L55 (19.7348, 32.9942) -> (19.7348, 9.7942)
  line L56 (-3.5, 31.5653) -> (-11, 31.5653)
  line L57 (-11, 31.5653) -> (-11, 11.5653)
  line L58 (-11, 11.5653) -> (-3.5, 11.5653)
  line L59 (-3.5, 11.5653) -> (-3.5, 31.5653)
  line L60 (-3.6, 31.4653) -> (-10.9, 31.4653)
  line L61 (-10.9, 31.4653) -> (-10.9, 11.6653)
  line L62 (-10.9, 11.6653) -> (-3.6, 11.6653)
  line L63 (-3.6, 11.6653) -> (-3.6, 31.4653)
  line L64 (-3.6, 11.6653) -> (3.662, 11.6653)
  line L65 (3.662, 11.6653) -> (3.662, 31.4653)
  line L66 (3.662, 31.4653) -> (-3.6, 31.4653)
  line L67 (-3.6, 31.4653) -> (-3.6, 11.6653)
  line L68 (-10.0691, 30.3942) -> (19.7348, 30.3942)
  line L69 (19.7348, 12.3942) -> (-10.0691, 12.3942)
  line L70 (-10.0691, 12.3942) -> (-10.0691, 30.3942)
  line L71 (-3.5, 15.1109) -> (-3.6, 15.0695) construction
  line L72 (-3.6, 27.7189) -> (-3.5, 27.6775) construction
  line L73 (19.7348, 11.8942) -> (-10.5691, 11.8942)
  line L74 (-10.5691, 11.8942) -> (-10.5691, 30.8942)
  line L75 (-10.5691, 30.8942) -> (19.7348, 30.8942)
  line L76 (19.8248, 9.8942) -> (29.8248, 9.8942)
  line L77 (-1.438, 9.8942) -> (3.562, 9.8942)
  line L78 (3.562, 32.8942) -> (-1.438, 32.8942)
  line L79 (29.8248, 32.8942) -> (19.8248, 32.8942)
  line L80 (29.8248, 8.3942) -> (19.8248, 8.3942)
  line L81 (3.562, 8.3942) -> (-1.438, 8.3942)
  line L82 (-1.438, 34.3942) -> (3.562, 34.3942)
  line L83 (19.8248, 34.3942) -> (29.8248, 34.3942)
  line L84 (19.7348, 30.8942) -> (18.5348, 30.8942)
  line L85 (18.5348, 30.8942) -> (18.5348, 30.3942)
  line L86 (11.0061, 12.3942) -> (11.0061, 11.8942)
  line L87 (-4.1273, 12.3942) -> (-4.1273, 11.8942)
  line L88 (-3.9549, 30.3942) -> (-3.9549, 30.8942)
  line L89 (31.5, 4) -> (46.5, 4)
  line L90 (46.5, 4) -> (84, 4)
  dimension "d262" = 0.1
  dimension "d263" = 0.1
  dimension "d264" = 20
  dimension "d265" = -0.1
  dimension "d272" = -0.5
  dimension "d303" = 1.2
  constraint horizontal L36
  constraint vertical L37
  constraint horizontal L38
  constraint vertical L39
  constraint coincident L30.start L38.start
  constraint horizontal L44
  constraint vertical L45
  constraint horizontal L46
  constraint vertical L47
  constraint coincident L13 L45.end
  constraint coincident L34.start L44.start
  constraint horizontal L52
  constraint vertical L53
  constraint horizontal L54
  constraint vertical L55
  constraint horizontal L56
  constraint vertical L57
  constraint horizontal L58
  constraint vertical L59
  constraint coincident L7 L56.start
  constraint horizontal L64
  constraint vertical L65
  constraint horizontal L66
  constraint vertical L67
  constraint coincident L53 L65.end
  constraint horizontal L68
  constraint parallel L68 L69
  constraint coincident L55 L69.start
  constraint coincident L55 L68.end
  constraint coincident L6 L71.start
  constraint coincident L7 L72.end
  constraint coincident L63 L71.end
  constraint coincident L63 L72.start
  constraint perpendicular L55 L84
  constraint coincident L68 L85.end
  constraint perpendicular L68 L85
  constraint coincident L69 L86.start
  constraint coincident L73 L86.end
  constraint perpendicular L73 L86
  constraint coincident L69 L87.start
  constraint coincident L73 L87.end
  constraint perpendicular L73 L87
  constraint coincident L68 L88.start
  constraint coincident L75 L88.end
  constraint perpendicular L75 L88
  measures "d264" distance of L56.start L58.end
  measures "d303" distance of L75.end L84.end
extrude "Extrude37" add sketch "Sketch7" along normal blind 6 separate body contours L4 L40 L41 L42 L52 | L4 L40 L42 L43 | L60 L61 L62 L63 L67 L73 L74 L75 | L63 L67 L69 L73 L87 | L63 L67 L68 L69 L70 | L68 L69 L70 L73 L74 L75 L87 L88 | L63 L67 L68 L75 L88 | L8 L48 L50 L51 | L8 L48 L49 L50 L54 makes body 16 at (14.3772, -4.1, 14) makes body 17 at (-6.0333, -18.2653, 16) makes body 18 at (9.0163, -35.2961, 16)
extrude "Extrude38" add sketch "Sketch7" along normal blind 1 from surface at 6 contours L4 L40 L41 L42 L52 | L4 L40 L42 L43 | L38 L41 L52 L53 L55 | L5 L59 L63 L64 L67 L73 | L5 L53 L59 L64 L65 L73 | L38 L53 L55 L65 L73 | L5 L59 L63 L67 L69 L73 | L5 L53 L59 L65 L69 L73 | L60 L61 L62 L63 L67 L73 L74 L75 | L5 L6 L7 L59 L63 L67 L68 L69 | L5 L6 L7 L53 L59 L65 L68 L69 | L53 L65 L69 L73 L86 | L63 L67 L69 L73 L87 | L55 L69 L73 L86 | L53 L55 L65 L68 L69 | L63 L67 L68 L69 L70 | L68 L69 L70 L73 L74 L75 L87 L88 | L7 L53 L59 L65 L66 L75 | L7 L59 L63 L66 L67 L75 | L7 L53 L59 L65 L68 L75 | L53 L65 L68 L75 L85 | L63 L67 L68 L75 L88 | L7 L59 L63 L67 L68 L75 | L44 L53 L55 L65 L75 L84 | L55 L68 L75 L84 L85 | L8 L48 L50 L51 | L8 L48 L49 L50 L54 | L44 L49 L53 L54 L55 bodies 16 17 18
chamfer "Chamfer7" distance 5.5 angle 45 2 edges at (3.662, -36.4471, 16) (3.662, -6.9471, 16) on bodies 16
chamfer "Chamfer8" distance 7 angle 45 2 edges at (3.662, -39.9, 9.75) (3.662, -4.1, 9.75) on bodies 16